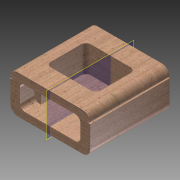
# Autodesk Inventor part: Motor Passenger Section
Saved by Autodesk Inventor 2015 (Build 190159000, 159)
## iProperties
Created: 2012-02-21
Part Number: Motor Passenger Section
Material: Generic
Document SubType Name: Modeling
Designer: Thom Tremblay
Density: 1 g/cm^3
Appearance: Cherry - Natural Low Gloss
Author: Thom Tremblay
Autodesk Inventor part; units mm, degrees
ref_plane "XZ Plane" through (0, 0, 0) normal (0, 1, 0) x (-1, 0, 0)
ref_plane "XY Plane" through (0, 0, 0) normal (0, 0, 1) x (1, 0, 0)
sketch "Sketch1" plane through (0, 0, 0) normal (0, 1, 0) x (-1, 0, 0)
  line L0 (-40.259, 19.431) -> (40.259, 19.431)
  line L1 (40.259, 19.431) -> (40.259, -19.431)
  line L2 (40.259, -19.431) -> (-40.259, -19.431)
  line L3 (-40.259, -19.431) -> (-40.259, 19.431)
  line L4 (-40.259, 11.811) -> (-38.735, 11.811)
  line L5 (-38.735, 11.811) -> (-38.735, 10.287)
  line L6 (-38.735, 10.287) -> (-40.259, 10.287)
  line L7 (-40.259, 10.287) -> (-40.259, 11.811)
  line L8 (40.259, 11.811) -> (38.735, 11.811)
  line L9 (38.735, 11.811) -> (38.735, 10.287)
  line L10 (38.735, 10.287) -> (40.259, 10.287)
  line L11 (40.259, 10.287) -> (40.259, 11.811)
  point P0 (0, 0)
  point P1 (40.259, 0)
  point P2 (0, -19.431)
  point P3 (0, 0)
  dimension "d0" = 80.518
  dimension "d1" = 38.862
  dimension "d20" = 1.524
  dimension "d21" = 7.62
  constraints: 24 end point, 6 parallel, 3 equal length, 3 horizontal, 3 perpendicular, 2 midpoint, 2 point on line, 1 coincident, 1 collinear, 1 horizontal alignment, 1 vertical alignment
  measures "d0" distance of L1.end L2.end
  measures "d1" distance of L0.end L1.end
  measures "d20" distance of L8.start L8.end
  measures "d21" distance between parallel lines of L0 L8
extrude "Extrusion1" add sketch "Sketch1" against normal blind 80.518 contours L0 L1 L8 L9 L10 L2 L3 L6 L5 L4
sketch "Sketch2" plane through (0, 0, 0) normal (0, 1, 0) x (-1, 0, 0)
  line L0 (-30.48, -11.811) -> (30.48, -11.811)
  line L1 (30.48, -11.811) -> (30.48, 11.811)
  line L2 (30.48, 11.811) -> (-30.48, 11.811)
  line L3 (-30.48, 11.811) -> (-30.48, -11.811)
  line L4 (40.259, -19.431) -> (-40.259, -19.431) projected
  line L5 (-40.259, 19.431) -> (40.259, 19.431) projected
  point P0 (0, 0)
  point P1 (0, 11.811)
  point P2 (-30.48, 0)
  dimension "d4" = 60.96
  dimension "d5" = 23.622
  constraints: 8 end point, 2 midpoint, 2 parallel, 1 horizontal, 1 horizontal alignment, 1 perpendicular, 1 vertical alignment
  measures "d4" distance of L2.end L1.end
  measures "d5" distance of L0.end L1.end
extrude "Extrusion2" cut sketch "Sketch2" against normal blind 14.478
sketch "Sketch3" plane through (0, -80.518, 0) normal (0, -1, 0) x (1, 0, 0)
  line L0 (-31.75, -12.7) -> (31.75, -12.7)
  line L1 (31.75, -12.7) -> (31.75, 12.7)
  line L2 (31.75, 12.7) -> (-31.75, 12.7)
  line L3 (-31.75, 12.7) -> (-31.75, -12.7)
  point P0 (0, 0)
  point P1 (0, -12.7)
  point P2 (-31.75, 0)
  dimension "d10" = 63.5
  dimension "d11" = 25.4
  constraints: 8 end point, 2 midpoint, 2 parallel, 1 horizontal, 1 horizontal alignment, 1 perpendicular, 1 vertical alignment
  measures "d10" distance of L1.end L2.end
  measures "d11" distance of L2.end L0.start
extrude "Extrusion3" cut sketch "Sketch3" against normal blind 14.478
sketch "Sketch4" plane through (40.259, 0, 19.431) normal (0, 0, 1) x (-1, 0, 0)
  line L0 (65.3415, 20.828) -> (15.1765, 20.828)
  line L1 (15.1765, 20.828) -> (15.1765, 61.214)
  line L2 (15.1765, 61.214) -> (65.3415, 61.214)
  line L3 (65.3415, 61.214) -> (65.3415, 20.828)
  line L4 (0, 0) -> (80.518, 0) projected
  point P0 (40.259, 0)
  point P1 (40.259, 0)
  point P2 (40.259, 20.828)
  dimension "d15" = 20.828
  dimension "d16" = 40.386
  dimension "d17" = 50.165
  constraints: 8 end point, 2 midpoint, 2 parallel, 1 horizontal, 1 perpendicular, 1 vertical alignment
  measures "d15" distance from line of L0 point (40.259, 0)
  measures "d16" distance of L0.end L1.end
  measures "d17" distance of L1.end L2.end
extrude "Extrusion4" cut sketch "Sketch4" against normal blind 27.178
fillet "Fillet1" radius 5.08 12 edges at (30.48, -7.239, 11.811) (30.48, -7.239, -11.811) (-30.48, -7.239, -11.811) (-30.48, -7.239, 11.811) (-31.75, -73.279, -12.7) (-31.75, -73.279, 12.7) (31.75, -73.279, 12.7) (31.75, -73.279, -12.7) (-25.0825, -20.828, 5.842) (25.0825, -20.828, 5.842) (25.0825, -61.214, 5.842) (-25.0825, -61.214, 5.842)
fillet "Fillet1" radius 7.62 4 edges at (-40.259, -40.259, 19.431) (-40.259, -40.259, -19.431) (40.259, -40.259, 19.431) (40.259, -40.259, -19.431)
fillet "Fillet2" radius 0.254 20 edges at (38.0272, -80.518, -17.1992) (0, -80.518, -19.431) (-38.0272, -80.518, -17.1992) (-40.259, -80.518, -0.7621) (40.259, -80.518, -0.7621) (0, -80.518, 19.431) (-38.0272, -80.518, 17.1992) (-40.259, -80.518, 11.8111) (38.0272, -80.518, 17.1992) (40.259, -80.518, 11.8111) (0, 0, 19.431) (-38.0272, 0, 17.1992) (-40.259, 0, 11.8111) (38.0272, 0, 17.1992) (40.259, 0, 11.8111) (38.0272, 0, -17.1992) (0, 0, -19.431) (-38.0272, 0, -17.1992) (-40.259, 0, -0.7621) (40.259, 0, -0.7621)
sketch "Sketch6" plane through (0, -14.478, 0) normal (0, 1, 0) x (1, 0, 0)
  line L0 (0, 27.2034) -> (0, -27.2034) projected
  line L1 (23.749, -11.811) -> (-23.749, -11.811)
  line L2 (-23.749, -11.811) -> (-23.749, 11.811)
  line L3 (-23.749, 11.811) -> (23.749, 11.811)
  line L4 (23.749, 11.811) -> (23.749, -11.811)
  line L5 (40.259, -10.287) -> (40.259, 11.811) projected
  line L6 (-40.259, 11.811) -> (-40.259, -10.287) projected
  line L7 (32.639, 19.431) -> (-32.639, 19.431) projected
  line L8 (25.4, -11.811) -> (-25.4, -11.811) projected
  line L9 (-25.4, 11.811) -> (25.4, 11.811) projected
  point P0 (0, 0)
  dimension "d26" = 16.51
  dimension "d28" = 16.51
  dimension "d30" = 0
  dimension "d31" = 0
  constraints: 8 end point, 2 parallel, 1 horizontal, 1 perpendicular
  measures "d26" distance between parallel lines of L5 L4
  measures "d28" distance between parallel lines of L6 L2
  measures "d30" distance between parallel lines of L8 L1
  measures "d31" distance between parallel lines of L3 L9
extrude "Extrusion5" cut sketch "Sketch6" against normal blind 25.4
body "Solid1"
